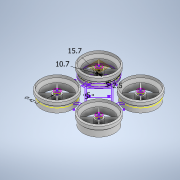
# Autodesk Inventor part: Main_Chassis
Saved by Autodesk Inventor 2021 (Build 250183000, 183)
## iProperties
Created: 2021-03-01
Part Number: Main_Chassis
Material: Generic
Document SubType Name: Modeling
Designer: Krutik
Density: 1 g/cm^3
Appearance: Default
Author: Krutik
Autodesk Inventor part; units mm, degrees
sketch "Sketch1" plane through (0, 0, 0) normal (0, 1, 0) x (-1, 0, 0)
  circle A0 centre (0, 0) radius 30
  arc A1 (16.9065, -18.4165) -> (18.4165, -16.9065) centre (0, 0) ccw
  line L0 (0, -1.51) -> (23.9095, -1.51) construction
  line L1 (0, 1.51) -> (23.9095, 1.51) construction
  arc A2 (-16.9065, 18.4165) -> (-18.4165, 16.9065) centre (0, 0) ccw
  arc A3 (-18.4165, -16.9065) -> (-16.9065, -18.4165) centre (0, 0) ccw
  arc A4 (16.9065, -18.4165) -> (18.4165, -16.9065) centre (0, 0) ccw
  arc A5 (18.4165, 16.9065) -> (16.9065, 18.4165) centre (0, 0) ccw
  arc A6 (18.4165, -16.9065) -> (18.4165, 16.9065) centre (0, 0) ccw
  arc A7 (16.9065, 18.4165) -> (-16.9065, 18.4165) centre (0, 0) ccw
  arc A8 (-18.4165, 16.9065) -> (-18.4165, -16.9065) centre (0, 0) ccw
  arc A9 (-16.9065, -18.4165) -> (16.9065, -18.4165) centre (0, 0) ccw
  circle A10 centre (0, 0) radius 5.35
  circle A11 centre (0, 0) radius 7.85
  line L2 (18.4165, 16.9065) -> (6.2542, 4.7442)
  line L3 (16.9065, 18.4165) -> (4.7442, 6.2542)
  line L4 (-16.9065, 18.4165) -> (-4.7442, 6.2542)
  line L5 (-6.2542, 4.7442) -> (-18.4165, 16.9065)
  line L6 (-6.2542, -4.7442) -> (-18.4165, -16.9065)
  line L7 (-16.9065, -18.4165) -> (-4.7442, -6.2542)
  line L8 (4.7442, -6.2542) -> (16.9065, -18.4165)
  line L9 (6.2542, -4.7442) -> (18.4165, -16.9065)
  point P0 (18.4165, -16.9065)
  point P1 (18.4165, -16.9065)
  dimension "d83" = 15.7
  dimension "d82" = 10.7
  constraints: 20 end point, 18 point on circle, 11 centre point, 7 coincident, 2 horizontal, 10 other
  measures "d82" diameter of A10
extrude "Extrusion3" add sketch "Sketch1" along normal blind 12.7 and the other way blind 3.7 contours A0
chamfer "Chamfer1" distance 4.8 angle 45 1 edges at (-17.6777, 12.7, -17.6777)
sketch "Sketch3" plane through (0, 12.7, 0) normal (0, 1, 0) x (1, 0, 0)
  circle A0 centre (0, 0) radius 2.875 projected
  circle A1 centre (0, 0) radius 29.8
  circle A2 centre (0, 0) radius 32
  point P0 (0, 0)
  dimension "d49" = 64
  constraints: 2 centre point, 2 coincident
  measures "d49" diameter of A2
ref_plane "Work Plane1" through (40, 0, 0) normal (1, 0, 0) x (0, 1, 0)
ref_plane "Work Plane2" through (0, 0, 40) normal (0, 0, 1) x (1, 0, 0)
mirror "Mirror1" about plane through (40, 0, 0) normal (1, 0, 0) of "Extrusion3", "Chamfer1"
mirror "Mirror3" about plane through (40, 0, 0) normal (1, 0, 0)
mirror "Mirror4" about plane through (0, 0, 40) normal (0, 0, 1) of "Extrusion3", "Chamfer1", "Mirror1"
ref_plane "Work Plane6" through (0, 5, 0) normal (0, 1, 0) x (-1, 0, 0)
extrude "Extrusion7" add sketch "Sketch3" along normal mid plane 10 contours A2
chamfer "Chamfer5" distance 2 angle 45 1 edges at (-32, 7.7, 0)
mirror "Mirror5" about plane through (0, 0, 40) normal (0, 0, 1) of "Extrusion7", "Chamfer5"
mirror "Mirror6" about plane through (40, 0, 0) normal (1, 0, 0) of "Extrusion7", "Chamfer5"
mirror "Mirror7" about plane through (40, 0, 0) normal (1, 0, 0) of "Mirror5"
extrude "Extrusion12" add sketch "Sketch1" along normal blind 7.9 and the other way blind 3.7 contours L8 A11 L9 A1 | A3 L6 A11 L7 | A11 | L2 A11 L3 A5 | A2 L4 A11 L5
mirror "Mirror8" about plane through (40, 0, 0) normal (1, 0, 0) of "Extrusion12"
mirror "Mirror9" about plane through (0, 0, 40) normal (0, 0, 1) of "Extrusion12"
mirror "Mirror10" about plane through (40, 0, 0) normal (1, 0, 0) of "Mirror9"
sketch "Sketch17" plane through (0, 5, 0) normal (0, 1, 0) x (-1, 0, 0)
  point P0 (0, 0)
chamfer "Chamfer9" distance 2.2 angle 45 4 edges at (112, 17.7, 0) (112, 17.7, 80) (-32, 17.7, 80) (-32, 17.7, 0)
sketch "Sketch22" plane through (0, 5, 0) normal (0, 1, 0) x (-1, 0, 0)
  circle A0 centre (-80, 80) radius 5.35 projected
  circle A1 centre (0, 80) radius 5.35 projected
  circle A2 centre (-80, 0) radius 5.35 projected
  circle A3 centre (0, 0) radius 5.35 projected
  circle A4 centre (0, 80) radius 29.8 projected
  circle A5 centre (0, 0) radius 29.8 projected
  arc A6 (-1.7319, 50.2504) -> (-5.1392, 29.3535) centre (7.6084, 38.0012) ccw
  arc A7 (-5.1392, 29.3535) -> (-6.3171, 29.1228) centre (0, 0) ccw
  arc A8 (-29.8, 0.0024) -> (-50.195, -0.0076) centre (-39.9936, -7.9098) ccw
  circle A9 centre (-80, 0) radius 5.35 projected
  arc A10 (-50.2002, 80) -> (-29.8003, 80) centre (-40.0002, 87.904) ccw
  arc A11 (-29.8003, 80) -> (-29.123, 73.683) centre (0, 80) ccw
  arc A12 (-50.8774, 73.683) -> (-50.2002, 80) centre (-80.0003, 80) ccw
  arc A13 (-79.9999, 29.8) -> (-79.9999, 50.2) centre (-87.9039, 40) ccw
  arc A14 (-73.6829, 29.1228) -> (-79.9999, 29.8) centre (-79.9999, 0) ccw
  arc A15 (-79.9999, 50.2) -> (-73.6829, 50.8772) centre (-79.9999, 80) ccw
  arc A16 (-73.6829, 29.1228) -> (-70.1753, 37.5) centre (-87.9039, 40) ccw
  arc A17 (-70.1753, 42.5) -> (-73.6829, 50.8772) centre (-87.9039, 40) ccw
  arc A18 (-50.8774, 73.683) -> (-41.25, 70.0437) centre (-40.0002, 87.904) ccw
  arc A19 (-38.75, 70.0438) -> (-29.123, 73.683) centre (-40.0002, 87.904) ccw
  line L0 (-28.3329, 51.6673) -> (-16.6656, 40.0001)
  line L1 (-16.6656, 40.0001) -> (-40, 16.6655)
  line L2 (-40, 16.6655) -> (-63.3346, 40)
  line L3 (-63.3346, 40) -> (-40.0002, 63.3345)
  line L4 (-40.0002, 63.3345) -> (-28.3329, 51.6673)
  line L5 (-39.9999, 13.1298) -> (-66.87, 39.9998)
  line L6 (-38.75, 66.87) -> (-38.75, 70.0438)
  line L7 (-38.75, 66.87) -> (-38.75, 65.62)
  line L8 (-41.25, 66.87) -> (-41.25, 70.0437)
  line L9 (-41.25, 66.87) -> (-41.25, 65.62)
  line L10 (-26.5651, 53.4351) -> (-38.75, 65.62)
  line L11 (-41.25, 65.62) -> (-66.87, 39.9998)
  line L12 (-13.1299, 38.75) -> (-9.9563, 38.75)
  line L13 (-13.1299, 38.75) -> (-14.3799, 38.75)
  line L14 (-13.1299, 41.25) -> (-9.9563, 41.25)
  line L15 (-13.1299, 41.25) -> (-14.3799, 41.25)
  line L16 (-26.5651, 53.4351) -> (-14.3799, 41.25)
  line L17 (-14.3799, 38.75) -> (-39.9999, 13.1298)
  arc A20 (-5.1392, 29.3535) -> (-4.7829, 29.4137) centre (0, 0) ccw
  arc A21 (-1.7319, 50.2504) -> (-1.7319, 50.2504) centre (0, 80) ccw
  line L18 (-9.9563, 38.75) -> (-7.4491, 38.75)
  line L19 (-9.9563, 41.25) -> (-7.4491, 41.25)
  arc A22 (-7.4491, 38.75) -> (-4.7829, 29.4137) centre (7.6084, 38.0012) ccw
  arc A23 (-1.7319, 50.2504) -> (-7.4491, 41.25) centre (7.6084, 38.0012) ccw
  line L20 (-40, 4.9942) -> (-40, 7.4942)
  arc A24 (-29.5985, 3.4579) -> (-40, 7.4942) centre (-39.9936, -7.9098) ccw
  circle A25 centre (-80, 0) radius 29.8 projected
  arc A26 (-40, 7.4942) -> (-50.4001, 3.4475) centre (-39.9936, -7.9098) ccw
  arc A27 (-29.6048, 3.4052) -> (-29.8, 0.0024) centre (0, 0) ccw
  point P0 (0, 0)
  point P1 (-29.1228, 73.6829)
  point P2 (-29.8, 80)
  point P3 (-50.8772, 73.6829)
  point P4 (-73.6829, 50.8772)
  point P5 (-50.8774, 73.683)
  dimension "d285" = 2.5
  constraints: 47 point on circle, 42 end point, 20 centre point, 11 coincident, 5 point on line, 4 horizontal, 4 perpendicular, 2 vertical, 1 concentric
  measures "d285" distance of L20.start L20.end
ref_plane "Work Plane7" through (0, 12.7, 0) normal (0, 1, 0) x (1, 0, 0)
sketch "Sketch23" plane through (0, 12.7, 0) normal (0, 1, 0) x (1, 0, 0)
  point P0 (0, 0)
ref_plane "Work Plane8" through (0, 12.7, 0) normal (0, 1, 0) x (1, 0, 0)
sketch "Sketch24" plane through (0, 12.7, 0) normal (0, 1, 0) x (1, 0, 0)
  circle A0 centre (0, 0) radius 5.35 projected
  circle A1 centre (80, -80) radius 5.35 projected
  circle A2 centre (80, 0) radius 5.35 projected
  circle A3 centre (0, -80) radius 5.35 projected
  line L0 (28.3327, -51.6673) -> (16.6655, -40)
  line L1 (16.6655, -40) -> (28.3327, -28.3327)
  line L2 (28.3327, -28.3327) -> (40, -16.6655)
  line L3 (40, -16.6655) -> (63.3345, -40)
  line L4 (63.3345, -40) -> (40, -63.3345)
  line L5 (40, -63.3345) -> (28.3327, -51.6673)
  line L6 (40, -63.3345) -> (36.4645, -59.799)
  line L7 (36.4645, -59.799) -> (40, -56.2635)
  line L8 (40, -56.2635) -> (43.5355, -59.799)
  circle A4 centre (40, -59.799) radius 1.5
  line L9 (16.6655, -40) -> (20.201, -43.5355)
  line L10 (20.201, -43.5355) -> (23.7365, -40)
  line L11 (23.7365, -40) -> (20.201, -36.4645)
  circle A5 centre (20.201, -40) radius 1.5
  line L12 (40, -16.6655) -> (36.4645, -20.201)
  line L13 (36.4645, -20.201) -> (40, -23.7365)
  line L14 (40, -23.7365) -> (43.5355, -20.201)
  circle A6 centre (40, -20.201) radius 1.5
  line L15 (63.3345, -40) -> (59.799, -43.5355)
  line L16 (59.799, -43.5355) -> (56.2635, -40)
  line L17 (56.2635, -40) -> (59.799, -36.4645)
  circle A7 centre (59.799, -40) radius 1.25
  point P0 (0, 0)
  dimension "d253" = 5
  dimension "d254" = 5
  dimension "d261" = 5
  dimension "d262" = 5
  constraints: 36 end point, 11 perpendicular, 9 point on line, 4 centre point
  measures "d253" distance of L4.end L6.end
  measures "d254" distance of L6.end L7.end
  measures "d261" distance of L2.end L12.end
  measures "d262" distance of L12.end L13.end
sketch "Sketch26" plane through (0, -3.7, 0) normal (0, -1, 0) x (1, 0, 0)
  circle A0 centre (0, 0) radius 5.35
  circle A1 centre (0, 80) radius 5.35 projected
  circle A2 centre (0, 80) radius 5.35
  circle A3 centre (80, 0) radius 5.35 projected
  circle A4 centre (80, 0) radius 5.35
  circle A5 centre (80, 80) radius 5.35 projected
  circle A6 centre (80, 80) radius 5.35
  arc A7 (58.0475, 20.1526) -> (58.0475, 20.1526) centre (80, 0) ccw projected
  circle A8 centre (78.35, -2.8579) radius 0.8
  circle A9 centre (78.35, 2.8579) radius 0.8
  circle A10 centre (83.3, 0) radius 0.8
  constraints: 7 centre point, 4 coincident
extrude "Extrusion21" add sketch "Sketch26" against normal blind 1 contours A3
mirror "Mirror11" about plane through (40, 0, 0) normal (1, 0, 0) of "Extrusion21"
mirror "Mirror12" about plane through (0, 0, 40) normal (0, 0, 1) of "Extrusion21"
mirror "Mirror13" about plane through (40, 0, 0) normal (1, 0, 0) of "Extrusion21", "Mirror12"
ref_plane "Work Plane4" through (80, 0, 40) normal (0, 0, -1) x (-1, 0, 0)
ref_plane "Work Plane5" through (40, 0, 80) normal (-1, 0, 0) x (0, 1, 0)
body "Solid2"
